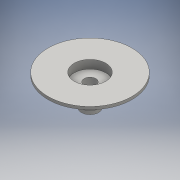
# Autodesk Inventor part: spool diam support
Saved by Autodesk Inventor 2016 SP1 (Build 200210100, 210)
## iProperties
Created: 2016-04-03
Part Number: spool diam support
Material: Generic
Document SubType Name: Modeling
Designer: ubik
Density: 1 g/cm^3
Appearance: Default
Author: ubik
Autodesk Inventor part; units mm, degrees
ref_plane "YZ Plane" through (0, 0, 0) normal (1, 0, 0) x (0, 1, 0)
ref_plane "XZ Plane" through (0, 0, 0) normal (0, 1, 0) x (-1, 0, 0)
ref_plane "XY Plane" through (0, 0, 0) normal (0, 0, 1) x (1, 0, 0)
sketch "Sketch1" plane through (0, 0, 0) normal (0, 0, 1) x (1, 0, 0)
  circle A0 centre (0, 0) radius 11.3
  circle A1 centre (0, 0) radius 30
  dimension "d0" = 22.6
  dimension "d1" = 60
  constraints: 2 centre point, 2 coincident
  measures "d0" diameter of A0
  measures "d1" diameter of A1
extrude "Extrusion1" add sketch "Sketch1" along normal blind 6
sketch "Sketch2" plane through (0, 0, 0) normal (1, 0, 0) x (0, 1, 0)
  line L0 (-30, 0) -> (30, 0) projected
  line L1 (0, 0) -> (0, -22.2563)
  line L2 (0, -28.8) -> (0, 4.8) projected
  line L3 (20.103, -4) -> (-2.6994, -4) construction
  line L4 (20.103, -8) -> (-2.6994, -8) construction
  line L5 (20.103, -12) -> (-2.6994, -12) construction
  line L6 (20.103, -16) -> (-2.6994, -16) construction
  line L7 (20.103, -20) -> (-2.6994, -20) construction
  line L8 (20.103, -24) -> (-2.6994, -24) construction
  line L9 (10.7198, -8) -> (10.7198, -4)
  line L10 (14.402, -4) -> (10.7198, -4)
  line L11 (8.1057, -12) -> (8.1057, -8)
  line L12 (10.7198, -8) -> (8.1057, -8)
  line L13 (6.0862, -16) -> (6.0862, -12)
  line L14 (8.1057, -12) -> (6.0862, -12)
  line L15 (6.0862, -16) -> (4.4759, -16)
  line L16 (14.402, -4) -> (14.402, 0)
  line L17 (4.4759, -16) -> (0, -16)
  point P0 (0, -11.3553)
  point P1 (0, -24)
  point P2 (0, -20)
  dimension "d8" = 4
  dimension "d11" = 4
  constraints: 32 end point, 16 point on line, 6 perpendicular, 2 collinear, 2 vertical, 1 parallel, 15 other
  measures "d8" distance between parallel lines of L0 L3
  measures "d11" distance of L3.start L4.start
revolve "Revolution1" add sketch "Sketch2" angle 360 about axis through (0, 0, -10) along (0, 0, 1)
sketch "Sketch3" plane through (0, 0, 0) normal (0, 0, 1) x (1, 0, 0)
  circle A0 centre (0, 0) radius 4.2
  dimension "d5" = 8.4
  constraints: 1 centre point, 1 coincident
  measures "d5" diameter of A0
extrude "Extrusion2" cut sketch "Sketch3" against normal through all
sketch "Sketch4" plane through (0, 0, 0) normal (0, 0, -1) x (-1, 0, 0)
  circle A0 centre (0, 0) radius 24
  circle A1 centre (0, 0) radius 30 projected
  dimension "d16" = 48
  constraints: 1 centre point, 1 coincident
  measures "d16" diameter of A0
extrude "Extrusion3" cut sketch "Sketch4" against normal blind 4
body "Solid1"
